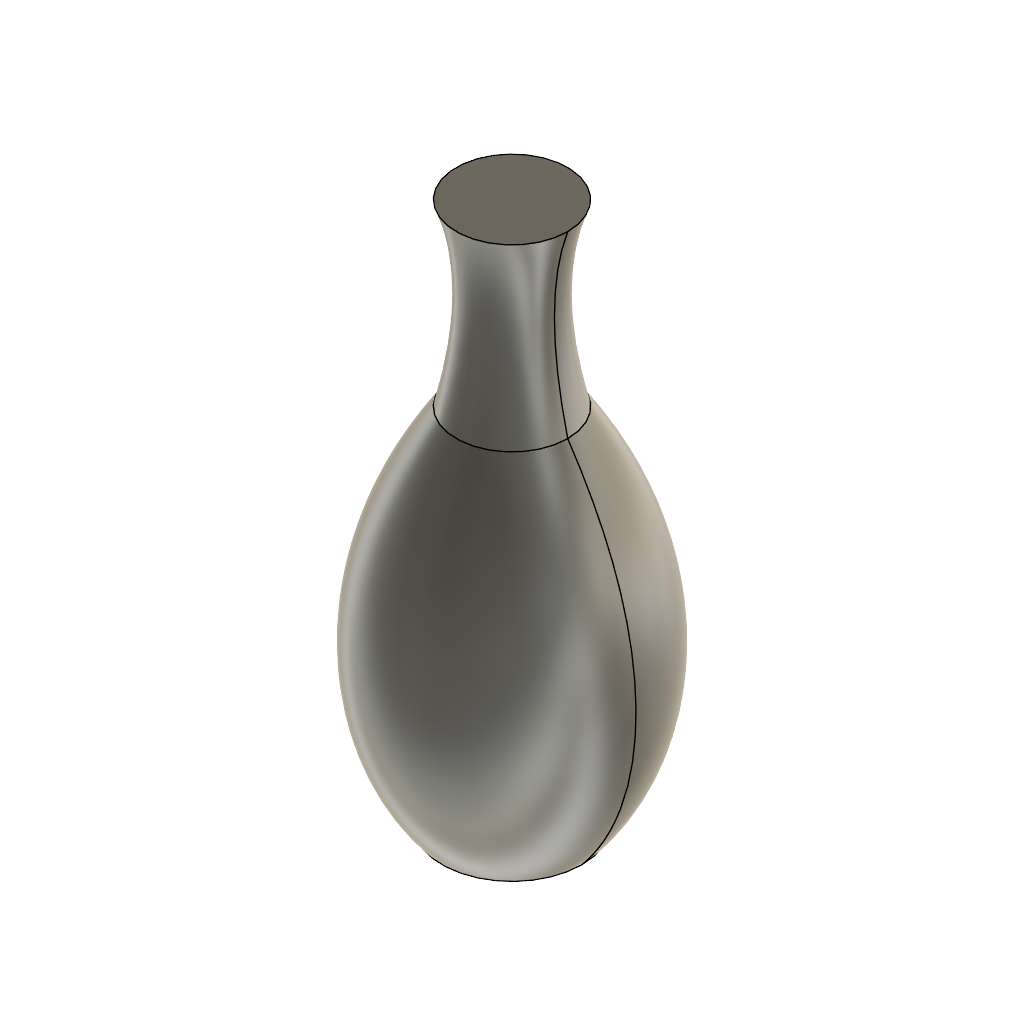
vase (Autodesk Fusion 360 design; units mm, degrees)
part number: 2026-09-27-13-22-59-727
Autodesk Fusion 360 part; units mm, degrees
sketch "草图2" plane through (0, 0, 0) normal (0, 1, 0) x (1, 0, 0)
  line L0 (0, 50) -> (25.0847, 50)
  line L1 (25.0847, 50) -> (50, 20) construction
  line L2 (50, 20) -> (50, -20) construction
  line L3 (50, -20) -> (40, -50) construction
  line L4 (40, -50) -> (20, -80) construction
  spline S0 degree 4 poles (25.0847, 50) (50, 20) (50, -20) (40, -50) (20, -80) knots 0 0 0 0 0 1 1 1 1 1
  line L5 (20, -80) -> (10.4482, -118.4632) construction
  line L6 (10.4482, -118.4632) -> (20, -144.363) construction
  spline S1 degree 2 poles (20, -80) (10.4482, -118.4632) (20, -144.363) knots 0 0 0 1 1 1
  line L7 (20, -144.363) -> (0, -144.363)
  line L8 (0, -144.363) -> (0, 50)
  constraint horizontal L0
  constraint horizontal L7
  constraint perpendicular L0 L8
revolve "旋转2" add sketch "草图2" angle 360 about axis through (0, 0, 144.363) along (0, 0, -1)
